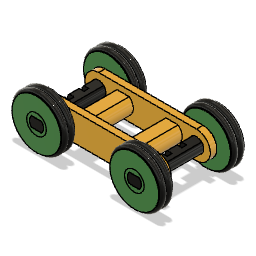
Rubber band car (Autodesk Fusion 360 design; units mm, degrees)
Autodesk Fusion 360 part; units mm, degrees
sketch "Sketch1" plane through (0, 0, 0) normal (0, 0, 1) x (1, 0, 0) in component "Chassis"
  circle A0 centre (-30, 0) radius 4.4375
  circle A1 centre (30, 0) radius 4.4375
  line L0 (-30, 8.4375) -> (30, 8.4375)
  line L1 (-30, -8.4375) -> (30, -8.4375)
  arc A2 (-30, 8.4375) -> (-30, -8.4375) centre (-30, 0) ccw
  arc A3 (30, -8.4375) -> (30, 8.4375) centre (30, 0) ccw
  line L2 (-12, 3) -> (-18, 3)
  line L3 (-18, -3) -> (-12, -3)
  line L4 (-12, 3) -> (-18, -3) construction
  line L5 (-18, 3) -> (-12, -3) construction
  arc A4 (-18, 3) -> (-18, -3) centre (-15, 0) ccw
  arc A5 (-12, -3) -> (-12, 3) centre (-15, 0) ccw
  line L6 (-18.7377, -5) -> (-11.2623, -5)
  arc A6 (-11.2623, -5) -> (-11.2623, 5) centre (-15, 0) ccw
  line L7 (-11.2623, 5) -> (-18.7377, 5)
  arc A7 (-18.7377, 5) -> (-18.7377, -5) centre (-15, 0) ccw
  line L8 (18.05, 3.05) -> (11.95, 3.05)
  line L9 (11.95, -3.05) -> (18.05, -3.05)
  line L10 (18.05, 3.05) -> (11.95, -3.05) construction
  line L11 (11.95, 3.05) -> (18.05, -3.05) construction
  arc A8 (11.95, 3.05) -> (11.95, -3.05) centre (15, 0) ccw
  arc A9 (18.05, -3.05) -> (18.05, 3.05) centre (15, 0) ccw
  point P0 (-15, 0)
  point P1 (15, 0)
  dimension "d1" = 8.875
  dimension "d2" = 8.875
  dimension "d5" = 6
  dimension "d6" = 6
  dimension "d7" = 2
  dimension "d8" = 6.1
  dimension "d9" = 6.1
  constraint tangent L0 A2
  constraint tangent L0 A3
  constraint horizontal L0
  constraint tangent L1 A3
  constraint parallel L0 L1
  constraint concentric A0 A2
  constraint concentric A1 A3
  constraint parallel L2 L3
  constraint horizontal L2
  constraint coincident L4 P0
  constraint coincident L5 P0
  constraint coincident P0 A4.centre
  constraint concentric A4 A5
  constraint parallel L8 L9
  constraint horizontal L8
  constraint coincident L10 P1
  constraint coincident L11 P1
  constraint coincident P1 A8.centre
  constraint concentric A8 A9
  measures "d1" diameter of A0
  measures "d2" diameter of A1
  measures "d5" distance of L3.start L3.end
  measures "d6" distance of L2.end L3.start
  measures "d8" distance of L9.start L9.end
  measures "d9" distance of L8.end L9.start
extrude "Extrude1" add sketch "Sketch1" against normal blind 4 contours L0 L1 A2 A3 makes body 1 in component "Chassis"
extrude "Extrude2" add sketch "Sketch1" against normal blind 28 contours L6 A6 L7 A7 bodies 1 in component "Chassis"
extrude "Extrude3" add sketch "Sketch1" against normal blind 32 contours L2 L3 A4 A5 bodies 1 in component "Chassis"
sketch "Sketch1 (2)" plane through (0, 0, 0) normal (0, 0, 1) x (1, 0, 0) in component "Axle"
  line L0 (-27, 3) -> (-33, 3)
  line L1 (-33, -3) -> (-27, -3)
  line L2 (-27, 3) -> (-33, -3) construction
  line L3 (-33, 3) -> (-27, -3) construction
  arc A0 (-33, 3) -> (-33, -3) centre (-30, 0) ccw
  arc A1 (-27, -3) -> (-27, 3) centre (-30, 0) ccw
  point P0 (-30, 0)
  dimension "d16" = 6
  dimension "d17" = 6
  constraint parallel L0 L1
  constraint horizontal L0
  constraint coincident L2 P0
  constraint coincident L3 P0
  constraint coincident P0 A0.centre
  constraint concentric A0 A1
  measures "d16" distance of L0.end L1.start
  measures "d17" distance of L1.start L1.end
extrude "Extrude1'" add sketch "Sketch1 (2)" along normal mid plane 52.2 separate body makes body 2 in component "Axle"
sketch "Sketch2" plane through (0, 0, 0) normal (0, 1, 0) x (1, 0, 0) in component "Axle"
  line L0 (-30, 3) -> (-36, 3)
  line L1 (-36, 3) -> (-36, -3)
  line L2 (-36, -3) -> (-30, -3)
  line L3 (-30, -3) -> (-30, 3)
  line L4 (-30, 3) -> (-36, -3) construction
  line L5 (-36, 3) -> (-30, -3) construction
  line L6 (-30, 6) -> (-39, 6)
  line L7 (-39, 6) -> (-39, -6)
  line L8 (-39, -6) -> (-30, -6)
  line L9 (-30, 3) -> (-30, 6)
  line L10 (-30, -3) -> (-30, -6)
  point P0 (-33, 0)
  dimension "d20" = 6
  dimension "d21" = 6
  dimension "d22" = 3
  constraint perpendicular L0 L1
  constraint parallel L0 L2
  constraint parallel L1 L3
  constraint horizontal L0
  constraint coincident L4 P0
  constraint coincident L5 P0
  measures "d20" distance of L0.end L1.end
  measures "d21" distance of L1.end L2.end
extrude "Extrude2'" cut sketch "Sketch2" along normal mid plane 8 contours L0 L1 L2 L6 L7 L8 L9 L10 bodies 2 in component "Axle"
sketch "Sketch1 (3)" plane through (0, 0, 0) normal (0, 0, 1) x (1, 0, 0) in component "Wheel"
  line L0 (-26.9589, 3.1) -> (-33.0411, 3.1)
  arc A0 (-33.0411, 3.1) -> (-33.0411, -3.1) centre (-30, 0) ccw
  line L1 (-33.0411, -3.1) -> (-26.9589, -3.1)
  arc A1 (-26.9589, -3.1) -> (-26.9589, 3.1) centre (-30, 0) ccw
  circle A2 centre (-30, 0) radius 6
  circle A3 centre (-30, 0) radius 15
  dimension "d26" = 12
  dimension "d27" = 30
  constraint concentric A1 A2
  constraint concentric A0 A3
  measures "d26" diameter of A2
  measures "d27" diameter of A3
extrude "Extrude1''" add sketch "Sketch1 (3)" against normal blind 1.4 separate body contours A2 makes body 3 in component "Wheel"
extrude "Extrude2''" add sketch "Sketch1 (3)" along normal blind 8.3 separate body contours A3 makes body 4 in component "Wheel"
torus "TorusPrimitive1" add centre line diameter 30 section diameter 3.4 placed x (1, 0, 0) y (0, 1, 0) z (0, 0, 1) at (-30, 0, 8.3) separate body makes body 5 in component "Wheel"
move_body "Move1" bodies 5 to x (1, 0, 0) y (0, 1, 0) z (0, 0, 1) at (0, 0, -2.2) in component "Wheel"
torus "TorusPrimitive2" add centre line diameter 30 section diameter 3.4 placed x (-1, 0, 0) y (0, 1, 0) z (0, 0, -1) at (-30, 0, 0) separate body makes body 6 in component "Wheel"
move_body "Move2" bodies 6 to x (1, 0, 0) y (0, 1, 0) z (0, 0, 1) at (0, 0, 2.2) in component "Wheel"
combine "Combine1" operation cut target body 4 tool bodies 5 6 keep tools in component "Wheel"
move_face "OffsetFaces1" offset 8.3 1 faces at (-30.1495, -4.0611, 0) on bodies 3 in component "Wheel"
component "Chassis" placed x (1, 0, 0) y (0, 1, 0) z (0, 0, 1) at (0, 0, 16)
component "Chassis" placed x (-1, 0, 0) y (0, 1, 0) z (0, 0, -1) at (0, 0, -16)
component "Axle" placed x (1, 0, 0) y (0, 1, 0) z (0, 0, 1) at (0, 0, 0)
component "Axle" placed x (1, 0, 0) y (0, 1, 0) z (0, 0, 1) at (60, 0, 0)
component "Wheel" placed x (1, 0, 0) y (0, 1, 0) z (0, 0, 1) at (0, 0, 17.8)
component "Wheel" placed x (1, 0, 0) y (0, 1, 0) z (0, 0, 1) at (60, 0, 17.8)
component "Wheel" placed x (1, 0, 0) y (0, -1, 0) z (0, 0, -1) at (0, 0, -17.8)
component "Wheel" placed x (1, 0, 0) y (0, -1, 0) z (0, 0, -1) at (60, 0, -17.8)
named bodies: "O-Ring 1", "O-Ring 2"
